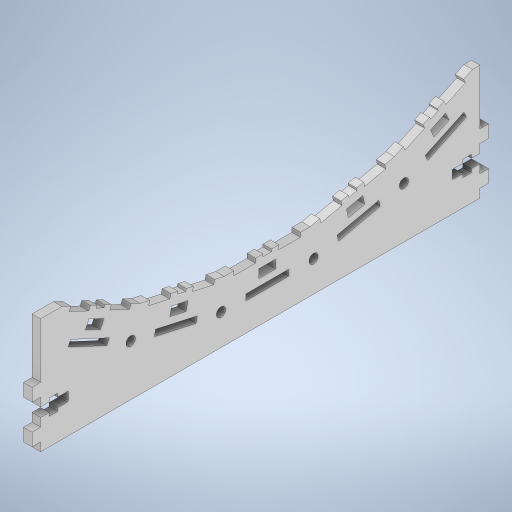
# Autodesk Inventor part: switchplate-support-05
Saved by Autodesk Inventor 2024.1 (Build 281209000, 209)
## iProperties
Created: 2019-06-27
Material: Acier, galvanisé
Document SubType Name: Modeling
Designer: Thibault
Density: 7.85 g/cm^3
Appearance: Aluminium - Poli
Mass: 11.7255 g
Surface Area: 33.7109 cm^2
Volume: 1.4937 cm^3
Part Number: switchplate-support-05
sa_0: 0.400 nd
height_shift: 0,000 mm
base_height: 27,000 mm
switchplate_depth: 107,000 mm
short_switchplate_depth: 86,200 mm
Author: Thibault
Autodesk Inventor part; units mm, degrees
ref_plane "YZ Plane" through (0, 0, 0) normal (1, 0, 0) x (0, 1, 0)
ref_plane "XZ Plane" through (0, 0, 0) normal (0, 1, 0) x (-1, 0, 0)
ref_plane "XY Plane" through (0, 0, 0) normal (0, 0, 1) x (1, 0, 0)
sketch "Anchor (nut side)" plane through (0, 0, 0) normal (0, 0, 1) x (1, 0, 0)
  line L0 (11.1, 0) -> (9.1, 0)
  line L1 (9.1, 0) -> (9.1, -2)
  line L2 (9.1, -2) -> (9.9, -2)
  line L3 (9.9, -2) -> (9.9, -4)
  line L4 (6.2, -4) -> (6.2, -2)
  line L5 (6.2, -2) -> (7, -2)
  line L6 (7, -2) -> (7, 0)
  line L7 (7, 0) -> (5, 0)
  line L8 (2, 0) -> (2, 2)
  line L9 (2, 0) -> (3, 0) construction
  line L10 (2, 2) -> (5, 2)
  line L11 (5, 2) -> (5, 0)
  line L12 (11.1, 0) -> (11.1, 2)
  line L13 (11.1, 2) -> (14.1, 2)
  line L14 (14.1, 2) -> (14.1, 0)
  line L15 (0, 0) -> (2, 0)
  line L16 (14.1, 0) -> (16.1, 0)
  line L17 (6.2, -4) -> (7, -4)
  line L18 (9.9, -4) -> (9.1, -4)
  line L19 (7, -4) -> (7, -6.25)
  line L20 (9.1, -4) -> (9.1, -6.25)
  line L21 (7.25, -6.5) -> (8.05, -6.5)
  arc A0 (7, -6.25) -> (7.25, -6.5) centre (7.25, -6.25) ccw
  arc A1 (8.85, -6.5) -> (9.1, -6.25) centre (8.85, -6.25) ccw
  line L22 (8.05, -6.5) -> (8.85, -6.5)
  line L23 (8.05, -3.8983) -> (8.05, -9.959) construction
  point P0 (9.1321, -0.6227)
  point P1 (7, -6.5)
  point P2 (9.1, -6.5)
  dimension "d3" = 2
  dimension "d7" = 6.1
  dimension "d10" = 2
  dimension "d11" = 2
  dimension "d12" = 0.8
  dimension "d13" = 2
  dimension "d14" = 0.8
  dimension "d15" = 2.1
  dimension "d18" = 2
  dimension "d19" = 0.8
  dimension "d20" = 0.8
  dimension "d21" = 2.5
  dimension "d22" = 2.5
  dimension "d23" = 2.1
  dimension "d38" = 2
  dimension "d39" = 0.25
  dimension "d120" = 3
  measures "d3" distance of point (0, 0) L8.start
  measures "d7" distance of L7.end L0.start
  measures "d10" distance of L0.start L0.end
  measures "d11" distance of L0.end L1.end
  measures "d12" distance of L1.end L2.end
  measures "d13" distance of L2.end L3.end
  measures "d14" distance of L4.end L5.end
  measures "d15" distance of L6.end L0.end
  measures "d18" distance of L14.end point (16.1, 0)
  measures "d19" distance of L4.start L17.end
  measures "d20" distance of L3.end L18.end
  measures "d21" distance of L17.end point (7, -6.5)
  measures "d22" distance of L18.end point (9.1, -6.5)
  measures "d23" distance of L17.end L18.end
  measures "d38" distance of the line from the sketch origin of L10
  measures "d39" radius of A0
  measures "d120" distance of L8.end L10.end
sketch "Anchor (screw side)" plane through (0, 0, 0) normal (0, 0, 1) x (1, 0, 0)
  circle A0 centre (93.8994, 50.2542) radius 1.05
  line L0 (90.8494, 51.2542) -> (87.8494, 51.2542)
  line L1 (87.8494, 51.2542) -> (87.8494, 49.2542)
  line L2 (87.8494, 49.2542) -> (90.8494, 49.2542)
  line L3 (90.8494, 49.2542) -> (90.8494, 51.2542)
  line L4 (99.9494, 51.2542) -> (96.9494, 51.2542)
  line L5 (96.9494, 51.2542) -> (96.9494, 49.2542)
  line L6 (96.9494, 49.2542) -> (99.9494, 49.2542)
  line L7 (99.9494, 49.2542) -> (99.9494, 51.2542)
  line L8 (90.8494, 51.2542) -> (96.9494, 49.2542) construction
  line L9 (96.9494, 51.2542) -> (90.8494, 49.2542) construction
  line L10 (85.8494, 53.2542) -> (101.9494, 53.2542) construction
  line L11 (101.9494, 53.2542) -> (101.9494, 47.2542) construction
  line L12 (101.9494, 47.2542) -> (85.8494, 47.2542) construction
  line L13 (85.8494, 47.2542) -> (85.8494, 53.2542) construction
  point P0 (103.5798, 50.1132)
  dimension "d27_1" = 2.1
  dimension "d28_1" = 3
  dimension "d29" = 2
  dimension "slot_distance" = 6.1
  dimension "d34" = 2
  dimension "d35" = 2
  dimension "d36" = 2
  dimension "d37" = 2
  measures "d27_1" diameter of A0
  measures "d28_1" distance of L2.end L1.end
  measures "d29" distance of L1.end L0.end
  measures "slot_distance" distance between parallel lines of L5 L3
  measures "d34" distance between parallel lines of L0 L10
  measures "d35" distance between parallel lines of L12 L2
  measures "d36" distance between parallel lines of L11 L7
  measures "d37" distance between parallel lines of L13 L1
sketch "Switch support" plane through (0, 0, 0) normal (0, 0, 1) x (1, 0, 0)
  line L0 (15.2854, 16.4472) -> (15.9854, 16.4472)
  line L1 (15.9854, 16.4472) -> (15.9854, 15.4472)
  line L2 (31.5854, 15.4472) -> (31.5854, 16.4472)
  line L3 (31.5854, 16.4472) -> (32.2854, 16.4472)
  line L4 (15.9854, 15.4472) -> (21.0554, 15.4472)
  line L5 (21.0554, 15.4472) -> (21.0554, 16.4472)
  line L6 (21.0554, 16.4472) -> (22.7854, 16.4472)
  line L7 (22.7854, 16.4472) -> (22.7854, 15.8972)
  line L8 (22.7854, 15.8972) -> (24.7854, 15.8972)
  line L9 (24.7854, 15.8972) -> (24.7854, 16.4472)
  line L10 (24.7854, 16.4472) -> (26.5154, 16.4472)
  line L11 (26.5154, 15.4472) -> (26.5154, 16.4472)
  line L12 (26.5154, 15.4472) -> (31.5854, 15.4472)
  line L13 (21.8354, 13.9472) -> (25.7354, 13.9472)
  line L14 (25.7354, 13.9472) -> (25.7354, 11.9472)
  line L15 (25.7354, 11.9472) -> (21.8354, 11.9472)
  line L16 (21.8354, 11.9472) -> (21.8354, 13.9472)
  line L17 (23.7854, 15.8972) -> (23.7854, 13.9472) construction
  line L18 (18.7854, 10.3472) -> (28.7854, 10.3472)
  line L19 (28.7854, 10.3472) -> (28.7854, 8.9472)
  line L20 (28.7854, 8.9472) -> (18.7854, 8.9472)
  line L21 (18.7854, 8.9472) -> (18.7854, 10.3472)
  line L22 (23.7854, 11.9472) -> (23.7854, 10.3472) construction
  point P0 (20.0288, 26.7181)
  point P1 (18.5204, 15.4472)
  dimension "d43" = 1
  dimension "d48" = 17
  dimension "d124" = 0.7
  dimension "d125" = 0.7
  dimension "d126" = 1
  dimension "d127" = 5.07
  dimension "d128" = 1
  dimension "d129" = 1.73
  dimension "d131" = 0.55
  dimension "d132" = 2
  dimension "d133" = 0.55
  dimension "d135" = 1.73
  dimension "d136" = 5.07
  dimension "d137" = 1
  dimension "d138" = 3.9
  dimension "d139" = 2
  dimension "d140" = 1.5
  dimension "d141" = 1.4
  dimension "d142" = 10
  dimension "d143" = 5.1
  measures "d43" distance of L1.start L1.end
  measures "d48" distance of point (32.285, 16.447) point (15.285, 16.447)
  measures "d124" distance of L2.end point (32.285, 16.447)
  measures "d125" distance of point (15.285, 16.447) L1.start
  measures "d126" distance of L2.start L2.end
  measures "d127" distance of L1.end L4.end
  measures "d128" distance of L4.end L5.end
  measures "d129" distance of L5.end L6.end
  measures "d131" distance of L6.end L7.end
  measures "d132" distance of L7.end L8.end
  measures "d133" distance of L8.end L9.end
  measures "d135" distance of L9.end L10.end
  measures "d136" distance of L11.start L2.start
  measures "d137" distance of L11.start L10.end
  measures "d138" distance of L14.end L15.end
  measures "d139" distance of L13.end L14.end
  measures "d140" distance between parallel lines of L13 L4
  measures "d141" distance of L20.end L18.start
  measures "d142" distance of L18.start L18.end
  measures "d143" distance from line of L18 point (18.52, 15.447)
sketch "Sketch1" plane through (0, 0, 0) normal (1, 0, 0) x (0, 1, 0)
  line L0 (0, -107) -> (27, -107)
  line L1 (27, 0) -> (0, 0)
  line L2 (27, -107) -> (27, -103.2572)
  line L3 (26.5066, -8.0581) -> (27, -7)
  line L4 (28.2121, -16.9724) -> (22.1003, -16.9724)
  line L5 (26.3238, -8.4501) -> (27, -7)
  line L6 (19.1393, -23.8573) -> (18.4631, -25.3074)
  line L7 (21.9473, -35.6102) -> (15.8356, -35.6102)
  line L8 (18.1168, -26.8695) -> (18.4631, -25.3074)
  line L9 (14.4373, -43.4665) -> (14.091, -45.0286)
  line L10 (19.8511, -55.1756) -> (13.7394, -55.1756)
  line L11 (14.091, -46.6286) -> (14.091, -45.0286)
  line L12 (14.091, -63.6286) -> (14.091, -65.2286)
  line L13 (22.0358, -74.7409) -> (15.9241, -74.7409)
  line L14 (14.4373, -66.7907) -> (14.091, -65.2286)
  line L15 (18.1168, -83.3877) -> (18.4631, -84.9498)
  line L16 (28.3566, -93.3787) -> (22.2449, -93.3787)
  line L17 (19.1393, -86.3999) -> (18.4631, -84.9498)
  line L18 (26.3238, -101.8071) -> (27, -103.2572)
  line L19 (27, 0) -> (27, -7)
  line L20 (0, 0) -> (0, -107)
  line L21 (13.8212, -17.5156) -> (10.037, -28.6632) construction
  line L22 (7.8727, -38.4262) -> (6.591, -50.1286) construction
  line L23 (13.8212, -92.7416) -> (10.037, -81.594) construction
  line L24 (6.591, -60.1286) -> (7.8727, -71.831) construction
  circle A0 centre (11.9291, -23.0894) radius 1.1
  circle A1 centre (7.2318, -44.2774) radius 1.1
  circle A2 centre (7.2318, -65.9798) radius 1.1
  circle A3 centre (11.9291, -87.1678) radius 1.1
  line L25 (18.1168, -26.8695) -> (17.9653, -27.5529)
  line L26 (17.9653, -27.5529) -> (16.989, -27.3365)
  line L27 (13.6125, -42.5667) -> (14.5888, -42.7831)
  line L28 (14.5888, -42.7831) -> (14.4373, -43.4665)
  line L29 (16.989, -27.3365) -> (15.8917, -32.2863)
  line L30 (15.8917, -32.2863) -> (16.868, -32.5027)
  line L31 (16.868, -32.5027) -> (16.4935, -34.1917)
  line L32 (16.4935, -34.1917) -> (15.9565, -34.0727)
  line L33 (15.9565, -34.0727) -> (15.5237, -36.0253)
  line L34 (15.5237, -36.0253) -> (16.0606, -36.1443)
  line L35 (16.0606, -36.1443) -> (15.6862, -37.8333)
  line L36 (14.7099, -37.6169) -> (15.6862, -37.8333)
  line L37 (14.7099, -37.6169) -> (13.6125, -42.5667)
  line L38 (14.2584, -32.7231) -> (13.4143, -36.5307)
  line L39 (13.4143, -36.5307) -> (11.4617, -36.0978)
  line L40 (11.4617, -36.0978) -> (12.3058, -32.2903)
  line L41 (12.3058, -32.2903) -> (14.2584, -32.7231)
  line L42 (15.7401, -35.049) -> (13.8363, -34.6269) construction
  line L43 (11.4039, -28.9662) -> (9.2395, -38.7292)
  line L44 (9.2395, -38.7292) -> (7.8727, -38.4262)
  line L45 (7.8727, -38.4262) -> (10.037, -28.6632)
  line L46 (10.037, -28.6632) -> (11.4039, -28.9662)
  line L47 (11.8837, -34.194) -> (10.3217, -33.8477) construction
  line L48 (26.3238, -8.4501) -> (26.028, -9.0845)
  line L49 (26.028, -9.0845) -> (25.1217, -8.6619)
  line L50 (18.5288, -22.8003) -> (19.4351, -23.2229)
  line L51 (19.4351, -23.2229) -> (19.1393, -23.8573)
  line L52 (25.1217, -8.6619) -> (22.979, -13.2569)
  line L53 (22.979, -13.2569) -> (23.8853, -13.6795)
  line L54 (23.8853, -13.6795) -> (23.1542, -15.2474)
  line L55 (23.1542, -15.2474) -> (22.6557, -15.015)
  line L56 (22.6557, -15.015) -> (21.8105, -16.8276)
  line L57 (21.8105, -16.8276) -> (22.3089, -17.06)
  line L58 (22.3089, -17.06) -> (21.5778, -18.6279)
  line L59 (20.6715, -18.2053) -> (21.5778, -18.6279)
  line L60 (20.6715, -18.2053) -> (18.5288, -22.8003)
  line L61 (21.2899, -13.3299) -> (19.6417, -16.8645)
  line L62 (19.6417, -16.8645) -> (17.8291, -16.0192)
  line L63 (17.8291, -16.0192) -> (19.4773, -12.4846)
  line L64 (19.4773, -12.4846) -> (21.2899, -13.3299)
  line L65 (22.2331, -15.9213) -> (20.4658, -15.0972) construction
  line L66 (19.3162, -9.0442) -> (15.09, -18.1073)
  line L67 (15.09, -18.1073) -> (13.8212, -17.5156)
  line L68 (13.8212, -17.5156) -> (18.0473, -8.4525)
  line L69 (18.0473, -8.4525) -> (19.3162, -9.0442)
  line L70 (18.6532, -14.2519) -> (17.2031, -13.5757) construction
  line L71 (14.091, -46.6286) -> (14.091, -47.3286)
  line L72 (14.091, -47.3286) -> (13.091, -47.3286)
  line L73 (13.091, -62.9286) -> (14.091, -62.9286)
  line L74 (14.091, -62.9286) -> (14.091, -63.6286)
  line L75 (13.091, -47.3286) -> (13.091, -52.3986)
  line L76 (13.091, -52.3986) -> (14.091, -52.3986)
  line L77 (14.091, -52.3986) -> (14.091, -54.1286)
  line L78 (14.091, -54.1286) -> (13.541, -54.1286)
  line L79 (13.541, -54.1286) -> (13.541, -56.1286)
  line L80 (13.541, -56.1286) -> (14.091, -56.1286)
  line L81 (14.091, -56.1286) -> (14.091, -57.8586)
  line L82 (13.091, -57.8586) -> (14.091, -57.8586)
  line L83 (13.091, -57.8586) -> (13.091, -62.9286)
  line L84 (11.591, -53.1786) -> (11.591, -57.0786)
  line L85 (11.591, -57.0786) -> (9.591, -57.0786)
  line L86 (9.591, -57.0786) -> (9.591, -53.1786)
  line L87 (9.591, -53.1786) -> (11.591, -53.1786)
  line L88 (13.541, -55.1286) -> (11.591, -55.1286) construction
  line L89 (7.991, -50.1286) -> (7.991, -60.1286)
  line L90 (7.991, -60.1286) -> (6.591, -60.1286)
  line L91 (6.591, -60.1286) -> (6.591, -50.1286)
  line L92 (6.591, -50.1286) -> (7.991, -50.1286)
  line L93 (9.591, -55.1286) -> (7.991, -55.1286) construction
  line L94 (14.4373, -66.7907) -> (14.5888, -67.4741)
  line L95 (14.5888, -67.4741) -> (13.6125, -67.6905)
  line L96 (16.989, -82.9207) -> (17.9653, -82.7043)
  line L97 (17.9653, -82.7043) -> (18.1168, -83.3877)
  line L98 (13.6125, -67.6905) -> (14.7099, -72.6403)
  line L99 (14.7099, -72.6403) -> (15.6862, -72.4239)
  line L100 (15.6862, -72.4239) -> (16.0606, -74.1129)
  line L101 (16.0606, -74.1129) -> (15.5237, -74.2319)
  line L102 (15.5237, -74.2319) -> (15.9565, -76.1845)
  line L103 (15.9565, -76.1845) -> (16.4935, -76.0655)
  line L104 (16.4935, -76.0655) -> (16.868, -77.7545)
  line L105 (15.8917, -77.9709) -> (16.868, -77.7545)
  line L106 (15.8917, -77.9709) -> (16.989, -82.9207)
  line L107 (13.4143, -73.7265) -> (14.2584, -77.5341)
  line L108 (14.2584, -77.5341) -> (12.3058, -77.9669)
  line L109 (12.3058, -77.9669) -> (11.4617, -74.1594)
  line L110 (11.4617, -74.1594) -> (13.4143, -73.7265)
  line L111 (15.7401, -75.2082) -> (13.8363, -75.6303) construction
  line L112 (9.2395, -71.528) -> (11.4039, -81.2909)
  line L113 (11.4039, -81.2909) -> (10.037, -81.594)
  line L114 (10.037, -81.594) -> (7.8727, -71.831)
  line L115 (7.8727, -71.831) -> (9.2395, -71.528)
  line L116 (11.8837, -76.0632) -> (10.3217, -76.4095) construction
  line L117 (19.1393, -86.3999) -> (19.4351, -87.0343)
  line L118 (19.4351, -87.0343) -> (18.5288, -87.4569)
  line L119 (25.1217, -101.5953) -> (26.028, -101.1727)
  line L120 (26.028, -101.1727) -> (26.3238, -101.8071)
  line L121 (18.5288, -87.4569) -> (20.6715, -92.0519)
  line L122 (20.6715, -92.0519) -> (21.5778, -91.6293)
  line L123 (21.5778, -91.6293) -> (22.3089, -93.1972)
  line L124 (22.3089, -93.1972) -> (21.8105, -93.4296)
  line L125 (21.8105, -93.4296) -> (22.6557, -95.2422)
  line L126 (22.6557, -95.2422) -> (23.1542, -95.0098)
  line L127 (23.1542, -95.0098) -> (23.8853, -96.5777)
  line L128 (22.979, -97.0003) -> (23.8853, -96.5777)
  line L129 (22.979, -97.0003) -> (25.1217, -101.5953)
  line L130 (19.6417, -93.3927) -> (21.2899, -96.9273)
  line L131 (21.2899, -96.9273) -> (19.4773, -97.7726)
  line L132 (19.4773, -97.7726) -> (17.8291, -94.238)
  line L133 (17.8291, -94.238) -> (19.6417, -93.3927)
  line L134 (22.2331, -94.3359) -> (20.4658, -95.16) construction
  line L135 (15.09, -92.1499) -> (19.3162, -101.213)
  line L136 (19.3162, -101.213) -> (18.0473, -101.8047)
  line L137 (18.0473, -101.8047) -> (13.8212, -92.7416)
  line L138 (13.8212, -92.7416) -> (15.09, -92.1499)
  line L139 (18.6532, -96.0053) -> (17.2031, -96.6815) construction
  point P0 (26.3238, -101.8071)
  point P1 (19.1393, -86.3999)
  point P2 (18.1168, -83.3877)
  point P3 (14.091, -63.6286)
  point P4 (14.4373, -43.4665)
  point P5 (18.1168, -26.8695)
  point P6 (26.3238, -8.4501)
  point P7 (0, -52.3792)
  point P8 (0, -17.4222)
  point P9 (22.6023, -16.9724)
  point P10 (22.9378, -16.9724)
  dimension "height" = 27
  dimension "d193" = 27
  dimension "k1_a" = 1.6
  dimension "k1_b" = 1.6
  dimension "k2_a" = 1.6
  dimension "k2_b" = 1.6
  dimension "k3_a" = 1.6
  dimension "k3_b" = 1.6
  dimension "k4_a" = 1.6
  dimension "k4_b" = 1.6
  dimension "k5_a" = 1.6
  dimension "k5_b" = 1.6
  dimension "d257" = 7
  dimension "d272" = 65
  dimension "d273" = 102.5
  dimension "d274" = 90
  dimension "d275" = 77.5
  dimension "d276" = 65
  dimension "d277" = 2.2
  dimension "d278" = 5.8862
  dimension "d279" = 5.8862
  dimension "d280" = 2.2
  dimension "d281" = 5.8862
  dimension "d282" = 5.8862
  dimension "d283" = 2.2
  dimension "d284" = 2.2
  constraints: 50 end point, 7 horizontal, 4 centre point, 4 midpoint, 4 vertical, 1 collinear, 1 vertical alignment, 27 other
  measures "height" distance of L1.start L1.end
  measures "d193" distance of L0.end L0.start
  measures "k1_a" distance of L3.end L5.start
  measures "k1_b" distance of L6.end L6.start
  measures "k2_a" distance of L8.start L6.end
  measures "k2_b" distance of L9.end L9.start
  measures "k3_a" distance of L11.start L9.end
  measures "k3_b" distance of L12.end L12.start
  measures "k4_a" distance of L14.start L12.end
  measures "k4_b" distance of L15.end L15.start
  measures "k5_a" distance of L17.start L15.end
  measures "k5_b" distance of L2.end L18.start
  measures "d257" distance of L1.start L3.end
  measures "d274" angle to the sketch y axis of L10
  measures "d277" diameter of A0
  measures "d280" diameter of A1
  measures "d283" diameter of A2
  measures "d284" diameter of A3
extrude "Base" add sketch "Sketch1" along normal blind 2
sketch "Sketch2" plane through (0, 0, 0) normal (-1, 0, 0) x (0, 0, 1)
  line L0 (-176.1228, 20.337) -> (-176.1228, -18.1383)
  line L1 (143.0949, 104.0572) -> (143.0949, -18.1383)
  line L2 (143.0949, -18.1383) -> (-176.1228, -18.1383)
  line L3 (-121, 0) -> (-121, 0) construction
  line L4 (-105, 16.1) -> (-105, 104.9044)
  line L5 (-105, 104.9044) -> (-176.1228, 104.9044)
  line L6 (-176.1228, 104.9044) -> (-176.1228, 20.337)
  line L7 (-2, 16.1) -> (-2, 104.0572)
  line L8 (-2, 104.0572) -> (143.0949, 104.0572)
  line L9 (0, 27) -> (0, 0) projected
  line L10 (-107, 0) -> (-107, 27) projected
  line L11 (0, 0) -> (-107, 0) projected
  line L12 (-2, 0) -> (-105, 0)
  line L13 (-105, 11.1) -> (-105, 9.1)
  line L14 (-105, 9.1) -> (-103, 9.1)
  line L15 (-103, 9.1) -> (-103, 9.9)
  line L16 (-103, 9.9) -> (-101, 9.9)
  line L17 (-101, 6.2) -> (-103, 6.2)
  line L18 (-103, 6.2) -> (-103, 7)
  line L19 (-103, 7) -> (-105, 7)
  line L20 (-105, 7) -> (-105, 5)
  line L21 (-105, 2) -> (-107, 2)
  line L22 (-105, 2) -> (-105, 3) construction
  line L23 (-107, 2) -> (-107, 5)
  line L24 (-107, 5) -> (-105, 5)
  line L25 (-105, 11.1) -> (-107, 11.1)
  line L26 (-107, 11.1) -> (-107, 14.1)
  line L27 (-107, 14.1) -> (-105, 14.1)
  line L28 (-105, 0) -> (-105, 2)
  line L29 (-105, 14.1) -> (-105, 16.1)
  line L30 (-101, 6.2) -> (-101, 7)
  line L31 (-101, 9.9) -> (-101, 9.1)
  line L32 (-101, 7) -> (-98.75, 7)
  line L33 (-101, 9.1) -> (-98.75, 9.1)
  line L34 (-98.5, 7.25) -> (-98.5, 8.05)
  arc A0 (-98.75, 7) -> (-98.5, 7.25) centre (-98.75, 7.25) ccw
  arc A1 (-98.5, 8.85) -> (-98.75, 9.1) centre (-98.75, 8.85) ccw
  line L35 (-98.5, 8.05) -> (-98.5, 8.85)
  line L36 (-101.1017, 8.05) -> (-95.041, 8.05) construction
  line L37 (-2, 5) -> (-2, 7)
  line L38 (-2, 7) -> (-4, 7)
  line L39 (-4, 7) -> (-4, 6.2)
  line L40 (-4, 6.2) -> (-6, 6.2)
  line L41 (-6, 9.9) -> (-4, 9.9)
  line L42 (-4, 9.9) -> (-4, 9.1)
  line L43 (-4, 9.1) -> (-2, 9.1)
  line L44 (-2, 9.1) -> (-2, 11.1)
  line L45 (-2, 14.1) -> (0, 14.1)
  line L46 (-2, 14.1) -> (-2, 13.1) construction
  line L47 (0, 14.1) -> (0, 11.1)
  line L48 (0, 11.1) -> (-2, 11.1)
  line L49 (-2, 5) -> (0, 5)
  line L50 (0, 5) -> (0, 2)
  line L51 (0, 2) -> (-2, 2)
  line L52 (-2, 16.1) -> (-2, 14.1)
  line L53 (-2, 2) -> (-2, 0)
  line L54 (-6, 9.9) -> (-6, 9.1)
  line L55 (-6, 6.2) -> (-6, 7)
  line L56 (-6, 9.1) -> (-8.25, 9.1)
  line L57 (-6, 7) -> (-8.25, 7)
  line L58 (-8.5, 8.85) -> (-8.5, 8.05)
  arc A2 (-8.25, 9.1) -> (-8.5, 8.85) centre (-8.25, 8.85) ccw
  arc A3 (-8.5, 7.25) -> (-8.25, 7) centre (-8.25, 7.25) ccw
  line L59 (-8.5, 8.05) -> (-8.5, 7.25)
  line L60 (-5.8983, 8.05) -> (-11.959, 8.05) construction
  point P0 (-2, 16.1)
  point P1 (-2, 0)
  point P2 (-105, 0)
  constraints: 20 end point, 3 horizontal, 3 vertical, 2 parallel, 1 perpendicular, 5 other
extrude "Standard anchors" cut sketch "Sketch2" against normal through all
sketch "Esquisse7" plane through (0, 0, 0) normal (-1, 0, 0) x (0, 0, 1)
  line L0 (-104.5, 8.35) -> (-102.5, 8.35) construction
  line L1 (-106.5, 9.15) -> (-104.5, 9.15) construction
  line L2 (-104.5, 5.85) -> (-106.5, 5.85) construction
  line L3 (-102.5, 6.65) -> (-104.5, 6.65) construction
  line L4 (-109, 9.15) -> (-100.5, 9.15)
  line L5 (-109, 5.85) -> (-100.5, 5.85)
  line L6 (-109, 10) -> (-109, 8.35) construction
  line L7 (-109, 9.15) -> (-109, 5.85)
  arc A0 (-102.5, 6.65) -> (-102.5, 8.35) centre (-102.5, 7.5) ccw projected
  line L8 (-100.5, 5.85) -> (-100.5, 9.15)
  point P0 (1.5, 20)
  point P1 (108.5, 20)
  point P2 (108.5, 0)
  point P3 (1.5, 0)
  point P4 (-2, 10)
  point P5 (-2, 5)
  point P6 (7.6691, 10.85)
  point P7 (8.8147, 9.7576)
  point P8 (-111, 0)
  point P9 (-102.77, 8.35)
  point P10 (-100.7609, 7.9198)
  dimension "d203" = 2
  constraints: 8 end point, 2 collinear, 1 perpendicular, 1 vertical, 2 other
  measures "d203" distance from line of L8 A0.centre
extrude "No back screw hole" [suppressed]
sketch "Esquisse8" plane through (0, 0, 0) normal (-1, 0, 0) x (0, 0, 1)
  line L0 (0, 0) -> (-100.5509, 0) projected
  line L1 (0, 0) -> (-20.4545, 0)
  line L2 (0, 67.0052) -> (0, 0)
  line L3 (0, 27) -> (0, 0) projected
  line L4 (-22.8003, 67.0052) -> (0, 67.0052)
  line L5 (-22.8003, 67.0052) -> (-22.8003, 16.1)
  line L6 (-107, 2) -> (-107, 27) projected
  line L7 (-22.8003, 5) -> (-22.8003, 7)
  line L8 (-22.8003, 7) -> (-24.8003, 7)
  line L9 (-24.8003, 7) -> (-24.8003, 6.2)
  line L10 (-24.8003, 6.2) -> (-26.8003, 6.2)
  line L11 (-26.8003, 9.9) -> (-24.8003, 9.9)
  line L12 (-24.8003, 9.9) -> (-24.8003, 9.1)
  line L13 (-24.8003, 9.1) -> (-22.8003, 9.1)
  line L14 (-22.8003, 9.1) -> (-22.8003, 11.1)
  line L15 (-22.8003, 14.1) -> (-20.8003, 14.1)
  line L16 (-22.8003, 14.1) -> (-22.8003, 13.1) construction
  line L17 (-20.8003, 14.1) -> (-20.8003, 11.1)
  line L18 (-20.8003, 11.1) -> (-22.8003, 11.1)
  line L19 (-22.8003, 5) -> (-20.8003, 5)
  line L20 (-20.8003, 5) -> (-20.8003, 2)
  line L21 (-20.8003, 2) -> (-22.8003, 2)
  line L22 (-22.8003, 16.1) -> (-22.8003, 14.1)
  line L23 (-22.8003, 2) -> (-22.8003, 0)
  line L24 (-26.8003, 9.9) -> (-26.8003, 9.1)
  line L25 (-26.8003, 6.2) -> (-26.8003, 7)
  line L26 (-26.8003, 9.1) -> (-29.0503, 9.1)
  line L27 (-26.8003, 7) -> (-29.0503, 7)
  line L28 (-29.3003, 8.85) -> (-29.3003, 8.05)
  arc A0 (-29.0503, 9.1) -> (-29.3003, 8.85) centre (-29.0503, 8.85) ccw
  arc A1 (-29.3003, 7.25) -> (-29.0503, 7) centre (-29.0503, 7.25) ccw
  line L29 (-29.3003, 8.05) -> (-29.3003, 7.25)
  line L30 (-26.6986, 8.05) -> (-32.7593, 8.05) construction
  point P0 (110, 0)
  point P1 (-109, 0)
  point P2 (-121, 0)
  point P3 (0, 12.75)
  point P4 (0, 10.25)
  point P5 (0, 12)
  point P6 (-22.8003, 0)
  point P7 (-107, 5)
  point P8 (-22.8003, 18.5288)
  dimension "d232" = 20.4545
  constraints: 8 end point, 2 collinear, 2 horizontal, 2 vertical, 1 parallel, 1 point on line, 2 other
  measures "d232" distance of L0.start L1.end
extrude "Short plate" [suppressed]
derived "shared_parameters.ipt"
equation "\"depth_shift\" = 3"
equation "\"angle\" = 12.5deg"
equation "\"a_default\" = 1.6"
equation "\"b_default\" = 1.6"
